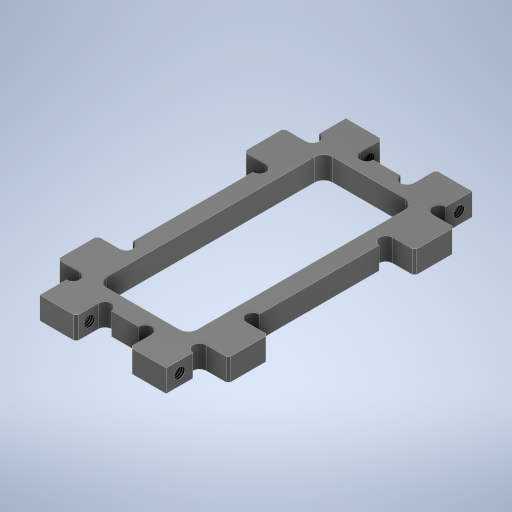
# Autodesk Inventor part: LegBaseBraceFrame
Saved by Autodesk Inventor 2024.2 (Build 282272000, 272)
## iProperties
Created: 2024-01-08
Part Number: LegBaseBraceFrame
Material: Acetal Resin, Black
Document SubType Name: Modeling
Designer: Masato Kubotera
Density: 1.425 g/cm^3
Appearance: Smooth - Black
Mass: 6.47212 g
Surface Area: 41.5244 cm^2
Volume: 4.54184 cm^3
Vendor: meviy
Author: Masato Kubotera
Autodesk Inventor part; units mm, degrees
ref_plane "YZ Plane" through (0, 0, 0) normal (1, 0, 0) x (0, 1, 0)
ref_plane "XZ Plane" through (0, 0, 0) normal (0, 1, 0) x (-1, 0, 0)
ref_plane "XY Plane" through (0, 0, 0) normal (0, 0, 1) x (1, 0, 0)
sketch "Sketch1" plane through (0, 0, 0) normal (0, 0, 1) x (1, 0, 0)
  line L0 (-55, -19.25) -> (14, -19.25)
  line L1 (14, -19.25) -> (14, 19.25)
  line L2 (14, 19.25) -> (-55, 19.25)
  line L3 (-55, 19.25) -> (-55, -19.25)
  line L4 (-55, -19.25) -> (14, 19.25) construction
  line L5 (14, -19.25) -> (-55, 19.25) construction
  line L6 (14, -6.05) -> (9, -6.05)
  line L7 (9, -6.05) -> (9, 6.05)
  line L8 (9, 6.05) -> (14, 6.05)
  line L9 (14, 0) -> (-55, 0)
  line L10 (-4, 14.25) -> (-37, 14.25)
  arc A0 (9, 6.05) -> (9, 3.05) centre (9, 4.55) ccw
  arc A1 (9, -3.05) -> (9, -6.05) centre (9, -4.55) ccw
  line L11 (-4, -14.25) -> (-37, -14.25)
  line L12 (-20.5, -19.25) -> (-20.5, 19.25) construction
  line L13 (-55, -6.05) -> (-50, -6.05)
  line L14 (-50, -6.05) -> (-50, 6.05)
  line L15 (-50, 6.05) -> (-55, 6.05)
  arc A2 (-50, 3.05) -> (-50, 6.05) centre (-50, 4.55) ccw
  arc A3 (-50, -6.05) -> (-50, -3.05) centre (-50, -4.55) ccw
  line L16 (5, -10.25) -> (5, 10.25)
  line L17 (5, 10.25) -> (-46, 10.25)
  line L18 (5, -10.25) -> (-46, -10.25)
  line L19 (-46, -10.25) -> (-46, 10.25)
  line L20 (-55, -14.25) -> (-46, -14.25)
  line L21 (-46, -14.25) -> (-46, -19.25)
  line L22 (-37, -19.25) -> (-37, -14.25)
  arc A4 (-46, -14.25) -> (-49, -14.25) centre (-47.5, -14.25) ccw
  arc A5 (-34, -14.25) -> (-37, -14.25) centre (-35.5, -14.25) ccw
  line L23 (-55, 14.25) -> (-46, 14.25)
  line L24 (-46, 14.25) -> (-46, 19.25)
  line L25 (-37, 19.25) -> (-37, 14.25)
  arc A6 (-49, 14.25) -> (-46, 14.25) centre (-47.5, 14.25) ccw
  arc A7 (-37, 14.25) -> (-34, 14.25) centre (-35.5, 14.25) ccw
  line L26 (-52, 14.25) -> (-52, 8.25) construction
  line L27 (14, 6) -> (9, 6) construction
  line L28 (14, -6) -> (9, -6) construction
  line L29 (-4, 19.25) -> (-4, 14.25)
  line L30 (14, 14.25) -> (5, 14.25)
  line L31 (5, 14.25) -> (5, 19.25)
  line L32 (11, 14.25) -> (11, 8.25) construction
  arc A8 (5, 14.25) -> (8, 14.25) centre (6.5, 14.25) ccw
  arc A9 (-7, 14.25) -> (-4, 14.25) centre (-5.5, 14.25) ccw
  line L33 (-4, -19.25) -> (-4, -14.25)
  line L34 (14, -14.25) -> (5, -14.25)
  line L35 (5, -14.25) -> (5, -19.25)
  arc A10 (8, -14.25) -> (5, -14.25) centre (6.5, -14.25) ccw
  arc A11 (-4, -14.25) -> (-7, -14.25) centre (-5.5, -14.25) ccw
  point P0 (0, 0)
  point P1 (-20.5, 0)
  point P2 (-55, 6.05)
  point P3 (-55, -6.05)
  point P4 (-37, 19.25)
  point P5 (-55, 14.25)
  point P6 (-34, 14.25)
  point P7 (5, 0)
  point P8 (9, 0)
  point P9 (-50, 0)
  point P10 (-46, 0)
  dimension "d0" = 38.5
  dimension "d2" = 12.1
  dimension "d3" = 14
  dimension "d4" = 5
  dimension "d12" = 1.5
  dimension "d27" = 69
  dimension "d36" = 2.5
  dimension "d40" = 9
  dimension "d42" = 6
  dimension "d51" = 2.5
  dimension "d55" = 12
  dimension "d56" = 0.05
  dimension "d57" = 5
  dimension "d58" = 9
  dimension "d59" = 6
  dimension "d70" = 9
  constraints: 72 end point, 38 symmetric about line, 27 point on line, 24 point on circle, 12 centre point, 8 vertical, 7 horizontal, 6 midpoint, 4 equal radius, 2 collinear, 2 parallel, 1 perpendicular, 1 tangent, 9 other
  measures "d0" distance of L0.end L1.end
  measures "d2" distance between parallel lines of L8 L6
  measures "d3" distance from line of L1 point (0, 0)
  measures "d4" distance of L7.end L8.end
  measures "d12" radius of A0
  measures "d27" distance between parallel lines of L1 L3
  measures "d36" distance edge to line of A0 L16
  measures "d40" distance between parallel lines of L24 L3
  measures "d42" distance of L26.start L26.end
  measures "d51" distance edge to line of A7 L17
  measures "d55" distance between parallel lines of L27 L28
  measures "d56" distance between parallel lines of L8 L27
  measures "d57" distance of L1.end L30.start
  measures "d58" distance between parallel lines of L1 L31
  measures "d59" distance of L32.start L32.end
  measures "d70" distance between parallel lines of L29 L31
extrude "Extrusion1" add sketch "Sketch1" along normal blind 5 contours L3 L23 A6 L24 L2 L25 A7 L10 A9 L29 L31 A8 L30 L1 L8 A0 L7 L9 L16 L17 L19 L14 A2 L15
fillet "Fillet1" radius 2 2 edges at (5, 10.25, 2.5) (-46, 10.25, 2.5)
sketch "Sketch5" plane through (-34, 14.25, 0) normal (0, 1, 0) x (1, 0, 0)
  line L0 (45, 0) -> (45, -5)
  line L1 (43, -5) -> (48, -5) projected
  line L2 (-18, 0) -> (-18, -5)
  line L3 (-15, -5) -> (-21, -5) projected
  point P0 (34, 0)
  point P1 (45, -2.5)
  point P2 (-18, -2.5)
  constraints: 4 end point, 3 midpoint, 2 vertical, 1 point on line
hole "Hole1" at (11, 14.25, 2.5) at (-52, 14.25, 2.5) direction (0, -1, 0) diameter 2.459 depth 8.8 thread size "M3x0.5" class "6H" standard "ANSI Metric M Profile"
chamfer "Chamfer1" distance 0.5 angle 45 6 edges at (14, 6.05, 2.5) (5, 19.25, 2.5) (-4, 19.25, 2.5) (-37, 19.25, 2.5) (-46, 19.25, 2.5) (-55, 6.05, 2.5)
mirror "Mirror1" about plane through (0, 0, 0) normal (0, 1, 0)
equation "\"d42\" = d6"
equation "\"d6\" = 6"
body "Solid1"
